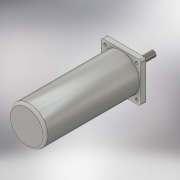
# Autodesk Inventor part: Nanotec-DH038-Servo-30W
Saved by Autodesk Inventor 2016 (Build 200138000, 138)
## iProperties
Created: 2015-05-16
Part Number: Nanotec-DH038-Servo-30W
Material: Generic
Document SubType Name: Modeling
Designer: as
Density: 1 g/cm^3
Appearance: Default
Mass: 117.901 g
Surface Area: 160.25 cm^2
Volume: 117.901 cm^3
Author: as
Autodesk Inventor part; units mm, degrees
ref_plane "YZ Plane" through (0, 0, 0) normal (1, 0, 0) x (0, 1, 0)
ref_plane "XZ Plane" through (0, 0, 0) normal (0, 1, 0) x (-1, 0, 0)
ref_plane "XY Plane" through (0, 0, 0) normal (0, 0, 1) x (1, 0, 0)
sketch "Sketch1" plane through (0, 0, 0) normal (0, 1, 0) x (-1, 0, 0)
  line L0 (20, 20) -> (-20, 20)
  line L1 (-20, 20) -> (-20, -20)
  line L2 (-20, -20) -> (20, -20)
  line L3 (20, -20) -> (20, 20)
  line L4 (20, 20) -> (-20, -20) construction
  line L5 (-20, 20) -> (20, -20) construction
  line L6 (16, 16) -> (-16, 16)
  line L7 (-16, 16) -> (-16, -16)
  line L8 (-16, -16) -> (16, -16)
  line L9 (16, -16) -> (16, 16)
  line L10 (16, 16) -> (-16, -16) construction
  line L11 (-16, 16) -> (16, -16) construction
  point P0 (0, 0)
  dimension "d0" = 40
  dimension "d1" = 40
  dimension "d2" = 32
  dimension "d3" = 32
  constraints: 24 end point, 4 coincident, 4 midpoint, 4 parallel, 2 horizontal, 2 perpendicular
  measures "d0" distance of L2.end L1.end
  measures "d1" distance of L0.end L1.end
  measures "d2" distance of L8.end L7.end
  measures "d3" distance of L6.end L7.end
extrude "Extrusion1" add sketch "Sketch1" along normal blind 5 contours L3 L2 L1 L0 | L9 L8 L7 L6
sketch "Sketch2" plane through (0, 5, 0) normal (0, 1, 0) x (1, 0, 0)
  circle A0 centre (0, 0) radius 15
  dimension "d7" = 30
  constraints: 1 centre point, 1 coincident
  measures "d7" diameter of A0
extrude "Extrusion2" add sketch "Sketch2" along normal blind 2.5
sketch "Sketch3" plane through (0, 0, 0) normal (0, -1, 0) x (1, 0, 0)
  circle A0 centre (0, 0) radius 19
  dimension "d10" = 38
  constraints: 1 centre point, 1 coincident
  measures "d10" diameter of A0
extrude "Extrusion3" add sketch "Sketch3" along normal blind 95
fillet "Fillet1" radius 2.5 1 edges at (-19, -95, 0)
fillet "Fillet2" radius 2 4 edges at (20, 2.5, -20) (-20, 2.5, -20) (-20, 2.5, 20) (20, 2.5, 20)
hole "Hole1" at (16, 0, -16) at (16, 0, 16) at (-16, 0, -16) at (-16, 0, 16) direction (0, 1, 0) diameter 3 depth 5 tip angle 118
sketch "Sketch4" plane through (0, 7.5, 0) normal (0, 1, 0) x (1, 0, 0)
  circle A0 centre (0, 0) radius 3
  dimension "d22" = 6
  constraints: 1 centre point, 1 coincident
  measures "d22" diameter of A0
extrude "Extrusion4" add sketch "Sketch4" along normal blind 25
equation "\"d1\" = d0"
equation "\"d3\" = d2"
body "Solid1"
